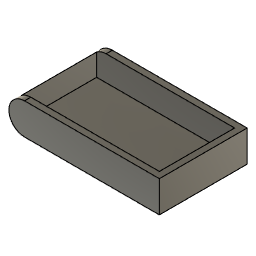
Controller Base (Autodesk Fusion 360 design; units mm, degrees)
Autodesk Fusion 360 part; units mm, degrees
note: some values were not read from the file. Chosen so that the rebuilt part matches the saved one: which face or edge a step refers to.
sketch "Sketch1" plane through (0, 0, 0) normal (0, 0, 1) x (1, 0, 0)
  line L0 (75, -25) -> (-45, -25)
  line L1 (-45, -25) -> (-45, 35)
  line L2 (-45, 35) -> (75, 35)
  line L3 (75, 35) -> (75, -25)
  constraint horizontal L0
  constraint vertical L1
  constraint horizontal L2
  constraint vertical L3
extrude "Extrude1" add sketch "Sketch1" along normal blind 5 and the other way blind 20
shell "Shell1" thickness 5 removed faces 1 at (-5, -5, 5)
move_face "MoveFace1" by (0, 5, 0) 2 faces at (-5, 35, -11.6667) (-3.3333, 30, -8.3333)
move_face "MoveFace2" by (0, -5, 0) 2 faces at (35, -25, -11.6667) (-3.3333, -20, -1.6667)
fillet "Fillet1" radius 12.5 2 edges at (-45, 5, 5) (-45, 5, -20)
